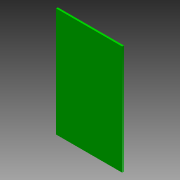
# Autodesk Inventor part: TableMount-Holder
Saved by Autodesk Inventor 2012 (Build 160160000, 160)
## iProperties
Created: 2013-07-16
Part Number: TableMount-Holder
Material: ABS Plastic
Document SubType Name: Modeling
Designer: joe_000
Density: 1.06 g/cm^3
Mass: 86.3684 g
Surface Area: 514.568 cm^2
Volume: 81.4797 cm^3
Author: joe_000
Autodesk Inventor part; units mm, degrees
ref_plane "YZ Plane" through (0, 0, 0) normal (1, 0, 0) x (0, 1, 0)
ref_plane "XZ Plane" through (0, 0, 0) normal (0, 1, 0) x (-1, 0, 0)
ref_plane "XY Plane" through (0, 0, 0) normal (0, 0, 1) x (1, 0, 0)
sketch "Sketch1" plane through (0, 0, 0) normal (0, 0, 1) x (1, 0, 0)
  line L0 (0, 0) -> (120, 0)
  line L1 (120, 0) -> (120, 198.5)
  line L2 (120, 198.5) -> (0, 198.5)
  line L3 (0, 198.5) -> (0, 0)
  dimension "d0" = 120
  dimension "d1" = 198.5
  constraints: 8 end point, 2 parallel, 1 horizontal, 1 perpendicular
  measures "d0" distance of L1.end L2.end
  measures "d1" distance of L0.end L1.end
extrude "Extrusion1" add sketch "Sketch1" along normal blind 3.175
equation "\"d0\" = TabletWidth"
equation "\"d1\" = TabletHeight"
equation "\"TabletWidth\" = 120"
equation "\"TabletHeight\" = 198.5"
body "Solid1"
